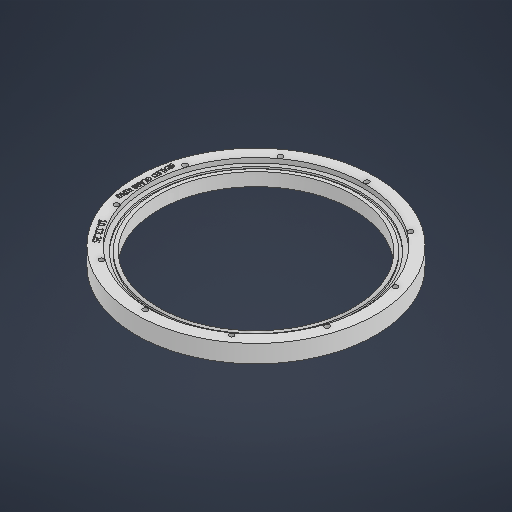
# Autodesk Inventor part: SealedGlassRing
Saved by Autodesk Inventor 2026.2 (Build 302298000, 298)
## iProperties
Created: 2025-06-19
Part Number: SealedGlassRing
Material: Generic
Document SubType Name: Modeling
Designer: mumin
Density: 1 g/cm^3
Appearance: Default
Author: mumin
Autodesk Inventor part; units mm, degrees
ref_plane "YZ Plane" through (0, 0, 0) normal (1, 0, 0) x (0, 1, 0)
ref_plane "XZ Plane" through (0, 0, 0) normal (0, 1, 0) x (-1, 0, 0)
ref_plane "XY Plane" through (0, 0, 0) normal (0, 0, 1) x (1, 0, 0)
sketch "Sketch1" plane through (0, 0, 0) normal (0, 1, 0) x (-1, 0, 0)
  circle A0 centre (0, 0) radius 110
  circle A1 centre (0, 0) radius 135
  dimension "d0" = 220
  dimension "d1" = 270
  constraints: 2 centre point, 2 coincident
  measures "d0" diameter of A0
  measures "d1" diameter of A1
extrude "Ring" add sketch "Sketch1" along normal blind 20
sketch "Sketch2" plane through (0, 20, 0) normal (0, 1, 0) x (1, 0, 0)
  circle A0 centre (0, 0) radius 122
  dimension "d4" = 244
  constraints: 1 centre point, 1 coincident
  measures "d4" diameter of A0
extrude "Glass Seat" cut sketch "Sketch2" against normal blind 5.3
sketch "Sketch3" plane through (0, 20, 0) normal (0, 1, 0) x (1, 0, 0)
  line L0 (0, 189) -> (0, -189) projected
  point P0 (0, 0)
  point P1 (0, 125)
  dimension "d14" = 125
  constraints: 1 point on line
  measures "d14" distance of point (0, 0) point (0, 125)
hole "Holes" at (0, 20, -125) direction (0, -1, 0) diameter 5.5 end through all
pattern_circular "Circular Pattern1" count 10 over 360 about axis through (0, -10, 0) along (0, 1, 0) of "Holes"
sketch "Sketch4" plane through (0, 20, 0) normal (0, 1, 0) x (1, 0, 0)
  line L0 (-123.4008, 33.078) -> (-123.4008, -40.8071) construction
  line L1 (-123.4008, -40.8071) -> (-126.5772, -40.8071) construction
  line L2 (-126.5772, -40.8071) -> (-126.5772, 33.078) construction
  line L3 (-126.5772, 33.078) -> (-123.4008, 33.078) construction
  spline S0 degree 2 poles (-128.5791, 31.1777) (-128.5791, 31.7207) (-128.3522, 32.4824) (-128.1901, 32.8187) knots 0 0 0 1 2 2 2
  line L4 (-128.1901, 32.8187) -> (-127.3554, 32.8187)
  line L5 (-127.3554, 32.8187) -> (-127.3554, 32.7701)
  spline S1 degree 2 poles (-127.3554, 32.7701) (-127.6634, 32.4419) (-128.0037, 31.6113) (-128.0037, 31.2263) knots 0 0 0 1 2 2 2
  spline S2 degree 2 poles (-128.0037, 31.2263) (-128.0037, 30.6753) (-127.5459, 30.1121) (-127.169, 30.1121) knots 0 0 0 1 2 2 2
  spline S3 degree 2 poles (-127.169, 30.1121) (-126.8692, 30.1121) (-126.4964, 30.4079) (-126.4032, 30.7279) knots 0 0 0 1 2 2 2
  spline S4 degree 2 poles (-126.4032, 30.7279) (-126.3384, 30.9589) (-126.2493, 31.3438) (-126.1763, 31.6315) knots 0 0 0 1 2 2 2
  spline S5 degree 2 poles (-126.1763, 31.6315) (-126.1074, 31.8908) (-125.9008, 32.3001) (-125.7347, 32.4581) knots 0 0 0 1 2 2 2
  spline S6 degree 2 poles (-125.7347, 32.4581) (-125.5685, 32.6121) (-125.1228, 32.7822) (-124.8311, 32.7822) knots 0 0 0 1 2 2 2
  spline S7 degree 2 poles (-124.8311, 32.7822) (-124.2233, 32.7822) (-123.4008, 31.8341) (-123.4008, 31.1007) knots 0 0 0 1 2 2 2
  spline S8 degree 2 poles (-123.4008, 31.1007) (-123.4008, 30.6793) (-123.5669, 29.9338) (-123.7249, 29.6137) knots 0 0 0 1 2 2 2
  line L6 (-123.7249, 29.6137) -> (-124.5191, 29.6137)
  line L7 (-124.5191, 29.6137) -> (-124.5191, 29.6623)
  spline S9 degree 2 poles (-124.5191, 29.6623) (-124.3003, 29.9014) (-123.9762, 30.6469) (-123.9762, 31.0561) knots 0 0 0 1 2 2 2
  spline S10 degree 2 poles (-123.9762, 31.0561) (-123.9762, 31.5181) (-124.4097, 32.0894) (-124.7622, 32.0894) knots 0 0 0 1 2 2 2
  spline S11 degree 2 poles (-124.7622, 32.0894) (-125.0783, 32.0894) (-125.4551, 31.7531) (-125.5402, 31.437) knots 0 0 0 1 2 2 2
  spline S12 degree 2 poles (-125.5402, 31.437) (-125.5969, 31.2263) (-125.7428, 30.6145) (-125.8036, 30.4119) knots 0 0 0 1 2 2 2
  spline S13 degree 2 poles (-125.8036, 30.4119) (-125.9616, 29.8973) (-126.5977, 29.4192) (-127.0637, 29.4192) knots 0 0 0 1 2 2 2
  spline S14 degree 2 poles (-127.0637, 29.4192) (-127.3595, 29.4192) (-127.9267, 29.6583) (-128.1253, 29.873) knots 0 0 0 1 2 2 2
  spline S15 degree 2 poles (-128.1253, 29.873) (-128.3441, 30.1121) (-128.5791, 30.7198) (-128.5791, 31.1777) knots 0 0 0 1 2 2 2
  line L8 (-128.4899, 28.7425) -> (-123.4899, 28.7425)
  line L9 (-123.4899, 28.7425) -> (-123.4899, 25.6145)
  line L10 (-123.4899, 25.6145) -> (-124.0815, 25.6145)
  line L11 (-124.0815, 25.6145) -> (-124.0815, 28.078)
  line L12 (-124.0815, 28.078) -> (-125.451, 28.078)
  line L13 (-125.451, 28.078) -> (-125.451, 25.7806)
  line L14 (-125.451, 25.7806) -> (-126.0426, 25.7806)
  line L15 (-126.0426, 25.7806) -> (-126.0426, 28.078)
  line L16 (-126.0426, 28.078) -> (-127.8984, 28.078)
  line L17 (-127.8984, 28.078) -> (-127.8984, 25.6145)
  line L18 (-127.8984, 25.6145) -> (-128.4899, 25.6145)
  line L19 (-128.4899, 25.6145) -> (-128.4899, 28.7425)
  line L20 (-128.4899, 25.4241) -> (-123.4899, 23.7385)
  line L21 (-123.4899, 23.7385) -> (-123.4899, 22.92)
  line L22 (-123.4899, 22.92) -> (-128.4899, 21.2344)
  line L23 (-128.4899, 21.2344) -> (-128.4899, 21.9354)
  line L24 (-128.4899, 21.9354) -> (-127.092, 22.3892)
  line L25 (-127.092, 22.3892) -> (-127.092, 24.2976)
  line L26 (-127.092, 24.2976) -> (-128.4899, 24.7514)
  line L27 (-128.4899, 24.7514) -> (-128.4899, 25.4241)
  line L28 (-126.5248, 22.5715) -> (-124.1707, 23.3455)
  line L29 (-124.1707, 23.3455) -> (-126.5248, 24.1153)
  line L30 (-126.5248, 24.1153) -> (-126.5248, 22.5715)
  line L31 (-128.4899, 17.8633) -> (-128.4899, 20.7604)
  line L32 (-128.4899, 20.7604) -> (-123.4899, 20.7604)
  line L33 (-123.4899, 20.7604) -> (-123.4899, 20.0959)
  line L34 (-123.4899, 20.0959) -> (-127.8984, 20.0959)
  line L35 (-127.8984, 20.0959) -> (-127.8984, 17.8633)
  line L36 (-127.8984, 17.8633) -> (-128.4899, 17.8633)
  line L37 (-128.4899, 17.3406) -> (-123.4899, 17.3406)
  line L38 (-123.4899, 17.3406) -> (-123.4899, 14.2126)
  line L39 (-123.4899, 14.2126) -> (-124.0815, 14.2126)
  line L40 (-124.0815, 14.2126) -> (-124.0815, 16.6761)
  line L41 (-124.0815, 16.6761) -> (-125.451, 16.6761)
  line L42 (-125.451, 16.6761) -> (-125.451, 14.3787)
  line L43 (-125.451, 14.3787) -> (-126.0426, 14.3787)
  line L44 (-126.0426, 14.3787) -> (-126.0426, 16.6761)
  line L45 (-126.0426, 16.6761) -> (-127.8984, 16.6761)
  line L46 (-127.8984, 16.6761) -> (-127.8984, 14.2126)
  line L47 (-127.8984, 14.2126) -> (-128.4899, 14.2126)
  line L48 (-128.4899, 14.2126) -> (-128.4899, 17.3406)
  spline S16 degree 2 poles (-125.994, 9.5408) (-126.6788, 9.5408) (-127.7809, 10.0959) (-128.0888, 10.5618) knots 0 0 0 1 2 2 2
  spline S17 degree 2 poles (-128.0888, 10.5618) (-128.3279, 10.9427) (-128.4899, 11.7247) (-128.4899, 12.3325) knots 0 0 0 1 2 2 2
  line L49 (-128.4899, 12.3325) -> (-128.4899, 13.4832)
  line L50 (-128.4899, 13.4832) -> (-123.4899, 13.4832)
  line L51 (-123.4899, 13.4832) -> (-123.4899, 12.3446)
  spline S18 degree 2 poles (-123.4899, 12.3446) (-123.4899, 11.6396) (-123.7006, 10.8373) (-123.887, 10.5537) knots 0 0 0 1 2 2 2
  spline S19 degree 2 poles (-123.887, 10.5537) (-124.2071, 10.0715) (-125.2647, 9.5408) (-125.994, 9.5408) knots 0 0 0 1 2 2 2
  spline S20 degree 2 poles (-125.9859, 10.2336) (-125.4105, 10.2336) (-124.5961, 10.6145) (-124.3651, 10.9913) knots 0 0 0 1 2 2 2
  spline S21 degree 2 poles (-124.3651, 10.9913) (-124.2071, 11.2587) (-124.0653, 11.8625) (-124.0653, 12.3122) knots 0 0 0 1 2 2 2
  line L52 (-124.0653, 12.3122) -> (-124.0653, 12.8187)
  line L53 (-124.0653, 12.8187) -> (-127.9146, 12.8187)
  line L54 (-127.9146, 12.8187) -> (-127.9146, 12.3122)
  spline S22 degree 2 poles (-127.9146, 12.3122) (-127.9146, 11.8706) (-127.7728, 11.202) (-127.5823, 10.9305) knots 0 0 0 1 2 2 2
  spline S23 degree 2 poles (-127.5823, 10.9305) (-127.3473, 10.5821) (-126.5694, 10.2336) (-125.9859, 10.2336) knots 0 0 0 1 2 2 2
  spline S24 degree 2 poles (-128.5872, 4.5772) (-128.5872, 5.108) (-128.263, 5.9873) (-127.9348, 6.3033) knots 0 0 0 1 2 2 2
  spline S25 degree 2 poles (-127.9348, 6.3033) (-127.6026, 6.6194) (-126.622, 6.9557) (-125.9859, 6.9557) knots 0 0 0 1 2 2 2
  spline S26 degree 2 poles (-125.9859, 6.9557) (-125.3822, 6.9557) (-124.4259, 6.6153) (-124.0856, 6.2993) knots 0 0 0 1 2 2 2
  spline S27 degree 2 poles (-124.0856, 6.2993) (-123.7574, 5.9954) (-123.4008, 5.104) (-123.4008, 4.5732) knots 0 0 0 1 2 2 2
  spline S28 degree 2 poles (-123.4008, 4.5732) (-123.4008, 4.3179) (-123.4737, 3.856) (-123.5386, 3.6453) knots 0 0 0 1 2 2 2
  spline S29 degree 2 poles (-123.5386, 3.6453) (-123.5872, 3.4751) (-123.7655, 3.0618) (-123.8303, 2.9362) knots 0 0 0 1 2 2 2
  line L55 (-123.8303, 2.9362) -> (-124.6326, 2.9362)
  line L56 (-124.6326, 2.9362) -> (-124.6326, 2.9929)
  spline S30 degree 2 poles (-124.6326, 2.9929) (-124.5232, 3.1185) (-124.3246, 3.3819) (-124.2112, 3.625) knots 0 0 0 1 2 2 2
  spline S31 degree 2 poles (-124.2112, 3.625) (-124.1099, 3.8276) (-123.9762, 4.3503) (-123.9762, 4.6502) knots 0 0 0 1 2 2 2
  spline S32 degree 2 poles (-123.9762, 4.6502) (-123.9762, 5.3714) (-125.0621, 6.2628) (-125.9656, 6.2628) knots 0 0 0 1 2 2 2
  spline S33 degree 2 poles (-125.9656, 6.2628) (-126.4681, 6.2628) (-127.2217, 6.0278) (-127.481, 5.8049) knots 0 0 0 1 2 2 2
  spline S34 degree 2 poles (-127.481, 5.8049) (-127.7403, 5.5902) (-128.0118, 4.9824) (-128.0118, 4.6015) knots 0 0 0 1 2 2 2
  spline S35 degree 2 poles (-128.0118, 4.6015) (-128.0118, 4.322) (-127.9308, 3.7628) (-127.8497, 3.5724) knots 0 0 0 1 2 2 2
  line L57 (-127.8497, 3.5724) -> (-126.5572, 3.5724)
  line L58 (-126.5572, 3.5724) -> (-126.5572, 4.7312)
  line L59 (-126.5572, 4.7312) -> (-125.9737, 4.7312)
  line L60 (-125.9737, 4.7312) -> (-125.9737, 2.916)
  line L61 (-125.9737, 2.916) -> (-128.1577, 2.916)
  spline S36 degree 2 poles (-128.1577, 2.916) (-128.2144, 3.0416) (-128.3886, 3.4711) (-128.4413, 3.6534) knots 0 0 0 1 2 2 2
  spline S37 degree 2 poles (-128.4413, 3.6534) (-128.5142, 3.9006) (-128.5872, 4.2976) (-128.5872, 4.5772) knots 0 0 0 1 2 2 2
  line L62 (-128.4899, -0.8158) -> (-128.4899, 2.0813)
  line L63 (-128.4899, 2.0813) -> (-123.4899, 2.0813)
  line L64 (-123.4899, 2.0813) -> (-123.4899, 1.4168)
  line L65 (-123.4899, 1.4168) -> (-127.8984, 1.4168)
  line L66 (-127.8984, 1.4168) -> (-127.8984, -0.8158)
  line L67 (-127.8984, -0.8158) -> (-128.4899, -0.8158)
  line L68 (-128.4899, -0.7996) -> (-123.4899, -2.4852)
  line L69 (-123.4899, -2.4852) -> (-123.4899, -3.3037)
  line L70 (-123.4899, -3.3037) -> (-128.4899, -4.9892)
  line L71 (-128.4899, -4.9892) -> (-128.4899, -4.2883)
  line L72 (-128.4899, -4.2883) -> (-127.092, -3.8345)
  line L73 (-127.092, -3.8345) -> (-127.092, -1.926)
  line L74 (-127.092, -1.926) -> (-128.4899, -1.4722)
  line L75 (-128.4899, -1.4722) -> (-128.4899, -0.7996)
  line L76 (-126.5248, -3.6521) -> (-124.1707, -2.8782)
  line L77 (-124.1707, -2.8782) -> (-126.5248, -2.1084)
  line L78 (-126.5248, -2.1084) -> (-126.5248, -3.6521)
  spline S38 degree 2 poles (-128.5791, -6.8571) (-128.5791, -6.3142) (-128.3522, -5.5524) (-128.1901, -5.2161) knots 0 0 0 1 2 2 2
  line L79 (-128.1901, -5.2161) -> (-127.3554, -5.2161)
  line L80 (-127.3554, -5.2161) -> (-127.3554, -5.2648)
  spline S39 degree 2 poles (-127.3554, -5.2648) (-127.6634, -5.593) (-128.0037, -6.4236) (-128.0037, -6.8085) knots 0 0 0 1 2 2 2
  spline S40 degree 2 poles (-128.0037, -6.8085) (-128.0037, -7.3596) (-127.5459, -7.9228) (-127.169, -7.9228) knots 0 0 0 1 2 2 2
  spline S41 degree 2 poles (-127.169, -7.9228) (-126.8692, -7.9228) (-126.4964, -7.627) (-126.4032, -7.3069) knots 0 0 0 1 2 2 2
  spline S42 degree 2 poles (-126.4032, -7.3069) (-126.3384, -7.0759) (-126.2493, -6.691) (-126.1763, -6.4033) knots 0 0 0 1 2 2 2
  spline S43 degree 2 poles (-126.1763, -6.4033) (-126.1074, -6.144) (-125.9008, -5.7348) (-125.7347, -5.5768) knots 0 0 0 1 2 2 2
  spline S44 degree 2 poles (-125.7347, -5.5768) (-125.5685, -5.4228) (-125.1228, -5.2526) (-124.8311, -5.2526) knots 0 0 0 1 2 2 2
  spline S45 degree 2 poles (-124.8311, -5.2526) (-124.2233, -5.2526) (-123.4008, -6.2007) (-123.4008, -6.9341) knots 0 0 0 1 2 2 2
  spline S46 degree 2 poles (-123.4008, -6.9341) (-123.4008, -7.3555) (-123.5669, -8.1011) (-123.7249, -8.4212) knots 0 0 0 1 2 2 2
  line L81 (-123.7249, -8.4212) -> (-124.5191, -8.4212)
  line L82 (-124.5191, -8.4212) -> (-124.5191, -8.3725)
  spline S47 degree 2 poles (-124.5191, -8.3725) (-124.3003, -8.1335) (-123.9762, -7.3879) (-123.9762, -6.9787) knots 0 0 0 1 2 2 2
  spline S48 degree 2 poles (-123.9762, -6.9787) (-123.9762, -6.5168) (-124.4097, -5.9455) (-124.7622, -5.9455) knots 0 0 0 1 2 2 2
  spline S49 degree 2 poles (-124.7622, -5.9455) (-125.0783, -5.9455) (-125.4551, -6.2818) (-125.5402, -6.5978) knots 0 0 0 1 2 2 2
  spline S50 degree 2 poles (-125.5402, -6.5978) (-125.5969, -6.8085) (-125.7428, -7.4203) (-125.8036, -7.6229) knots 0 0 0 1 2 2 2
  spline S51 degree 2 poles (-125.8036, -7.6229) (-125.9616, -8.1375) (-126.5977, -8.6156) (-127.0637, -8.6156) knots 0 0 0 1 2 2 2
  spline S52 degree 2 poles (-127.0637, -8.6156) (-127.3595, -8.6156) (-127.9267, -8.3766) (-128.1253, -8.1618) knots 0 0 0 1 2 2 2
  spline S53 degree 2 poles (-128.1253, -8.1618) (-128.3441, -7.9228) (-128.5791, -7.315) (-128.5791, -6.8571) knots 0 0 0 1 2 2 2
  spline S54 degree 2 poles (-128.5791, -10.6862) (-128.5791, -10.1432) (-128.3522, -9.3815) (-128.1901, -9.0451) knots 0 0 0 1 2 2 2
  line L83 (-128.1901, -9.0451) -> (-127.3554, -9.0451)
  line L84 (-127.3554, -9.0451) -> (-127.3554, -9.0938)
  spline S55 degree 2 poles (-127.3554, -9.0938) (-127.6634, -9.422) (-128.0037, -10.2526) (-128.0037, -10.6375) knots 0 0 0 1 2 2 2
  spline S56 degree 2 poles (-128.0037, -10.6375) (-128.0037, -11.1886) (-127.5459, -11.7518) (-127.169, -11.7518) knots 0 0 0 1 2 2 2
  spline S57 degree 2 poles (-127.169, -11.7518) (-126.8692, -11.7518) (-126.4964, -11.456) (-126.4032, -11.1359) knots 0 0 0 1 2 2 2
  spline S58 degree 2 poles (-126.4032, -11.1359) (-126.3384, -10.905) (-126.2493, -10.52) (-126.1763, -10.2323) knots 0 0 0 1 2 2 2
  spline S59 degree 2 poles (-126.1763, -10.2323) (-126.1074, -9.973) (-125.9008, -9.5638) (-125.7347, -9.4058) knots 0 0 0 1 2 2 2
  spline S60 degree 2 poles (-125.7347, -9.4058) (-125.5685, -9.2518) (-125.1228, -9.0816) (-124.8311, -9.0816) knots 0 0 0 1 2 2 2
  spline S61 degree 2 poles (-124.8311, -9.0816) (-124.2233, -9.0816) (-123.4008, -10.0298) (-123.4008, -10.7631) knots 0 0 0 1 2 2 2
  spline S62 degree 2 poles (-123.4008, -10.7631) (-123.4008, -11.1845) (-123.5669, -11.9301) (-123.7249, -12.2502) knots 0 0 0 1 2 2 2
  line L85 (-123.7249, -12.2502) -> (-124.5191, -12.2502)
  line L86 (-124.5191, -12.2502) -> (-124.5191, -12.2015)
  spline S63 degree 2 poles (-124.5191, -12.2015) (-124.3003, -11.9625) (-123.9762, -11.2169) (-123.9762, -10.8077) knots 0 0 0 1 2 2 2
  spline S64 degree 2 poles (-123.9762, -10.8077) (-123.9762, -10.3458) (-124.4097, -9.7745) (-124.7622, -9.7745) knots 0 0 0 1 2 2 2
  spline S65 degree 2 poles (-124.7622, -9.7745) (-125.0783, -9.7745) (-125.4551, -10.1108) (-125.5402, -10.4268) knots 0 0 0 1 2 2 2
  spline S66 degree 2 poles (-125.5402, -10.4268) (-125.5969, -10.6375) (-125.7428, -11.2494) (-125.8036, -11.452) knots 0 0 0 1 2 2 2
  spline S67 degree 2 poles (-125.8036, -11.452) (-125.9616, -11.9665) (-126.5977, -12.4447) (-127.0637, -12.4447) knots 0 0 0 1 2 2 2
  spline S68 degree 2 poles (-127.0637, -12.4447) (-127.3595, -12.4447) (-127.9267, -12.2056) (-128.1253, -11.9909) knots 0 0 0 1 2 2 2
  spline S69 degree 2 poles (-128.1253, -11.9909) (-128.3441, -11.7518) (-128.5791, -11.144) (-128.5791, -10.6862) knots 0 0 0 1 2 2 2
  line L87 (-128.4899, -19.1383) -> (-128.4899, -18.2753)
  line L88 (-128.4899, -18.2753) -> (-126.5005, -16.6951)
  line L89 (-126.5005, -16.6951) -> (-126.5005, -15.9333)
  line L90 (-126.5005, -15.9333) -> (-128.4899, -15.9333)
  line L91 (-128.4899, -15.9333) -> (-128.4899, -15.2688)
  line L92 (-128.4899, -15.2688) -> (-123.4899, -15.2688)
  line L93 (-123.4899, -15.2688) -> (-123.4899, -16.5573)
  spline S70 degree 2 poles (-123.4899, -16.5573) (-123.4899, -16.9868) (-123.5831, -17.5662) (-123.7533, -17.8296) knots 0 0 0 1 2 2 2
  spline S71 degree 2 poles (-123.7533, -17.8296) (-123.9235, -18.093) (-124.4543, -18.3968) (-124.8473, -18.3968) knots 0 0 0 1 2 2 2
  spline S72 degree 2 poles (-124.8473, -18.3968) (-125.3943, -18.3968) (-126.1358, -17.8377) (-126.3141, -17.3596) knots 0 0 0 1 2 2 2
  line L94 (-126.3141, -17.3596) -> (-128.4899, -19.1383)
  spline S73 degree 2 poles (-124.9, -17.704) (-124.6812, -17.704) (-124.3449, -17.55) (-124.2355, -17.3879) knots 0 0 0 1 2 2 2
  spline S74 degree 2 poles (-124.2355, -17.3879) (-124.1423, -17.2461) (-124.0653, -16.8693) (-124.0653, -16.5938) knots 0 0 0 1 2 2 2
  line L95 (-124.0653, -16.5938) -> (-124.0653, -15.9333)
  line L96 (-124.0653, -15.9333) -> (-125.9454, -15.9333)
  line L97 (-125.9454, -15.9333) -> (-125.9454, -16.5168)
  spline S75 degree 2 poles (-125.9454, -16.5168) (-125.9454, -16.8045) (-125.8441, -17.2623) (-125.686, -17.4203) knots 0 0 0 1 2 2 2
  spline S76 degree 2 poles (-125.686, -17.4203) (-125.5483, -17.5662) (-125.1593, -17.704) (-124.9, -17.704) knots 0 0 0 1 2 2 2
  line L98 (-128.4899, -21.2777) -> (-128.4899, -19.3409)
  line L99 (-128.4899, -19.3409) -> (-127.9794, -19.3409)
  line L100 (-127.9794, -19.3409) -> (-127.9794, -19.9771)
  line L101 (-127.9794, -19.9771) -> (-124.0005, -19.9771)
  line L102 (-124.0005, -19.9771) -> (-124.0005, -19.3409)
  line L103 (-124.0005, -19.3409) -> (-123.4899, -19.3409)
  line L104 (-123.4899, -19.3409) -> (-123.4899, -21.2777)
  line L105 (-123.4899, -21.2777) -> (-124.0005, -21.2777)
  line L106 (-124.0005, -21.2777) -> (-124.0005, -20.6416)
  line L107 (-124.0005, -20.6416) -> (-127.9794, -20.6416)
  line L108 (-127.9794, -20.6416) -> (-127.9794, -21.2777)
  line L109 (-127.9794, -21.2777) -> (-128.4899, -21.2777)
  line L110 (-128.4899, -25.678) -> (-128.4899, -24.9325)
  line L111 (-128.4899, -24.9325) -> (-124.1788, -22.7202)
  line L112 (-124.1788, -22.7202) -> (-128.4899, -22.7202)
  line L113 (-128.4899, -22.7202) -> (-128.4899, -22.1003)
  line L114 (-128.4899, -22.1003) -> (-123.4899, -22.1003)
  line L115 (-123.4899, -22.1003) -> (-123.4899, -23.0443)
  line L116 (-123.4899, -23.0443) -> (-127.4486, -25.0581)
  line L117 (-127.4486, -25.0581) -> (-123.4899, -25.0581)
  line L118 (-123.4899, -25.0581) -> (-123.4899, -25.678)
  line L119 (-123.4899, -25.678) -> (-128.4899, -25.678)
  spline S77 degree 2 poles (-128.5872, -28.7858) (-128.5872, -28.255) (-128.263, -27.3758) (-127.9348, -27.0597) knots 0 0 0 1 2 2 2
  spline S78 degree 2 poles (-127.9348, -27.0597) (-127.6026, -26.7437) (-126.622, -26.4074) (-125.9859, -26.4074) knots 0 0 0 1 2 2 2
  spline S79 degree 2 poles (-125.9859, -26.4074) (-125.3822, -26.4074) (-124.4259, -26.7477) (-124.0856, -27.0638) knots 0 0 0 1 2 2 2
  spline S80 degree 2 poles (-124.0856, -27.0638) (-123.7574, -27.3677) (-123.4008, -28.2591) (-123.4008, -28.7899) knots 0 0 0 1 2 2 2
  spline S81 degree 2 poles (-123.4008, -28.7899) (-123.4008, -29.0451) (-123.4737, -29.5071) (-123.5386, -29.7178) knots 0 0 0 1 2 2 2
  spline S82 degree 2 poles (-123.5386, -29.7178) (-123.5872, -29.8879) (-123.7655, -30.3012) (-123.8303, -30.4268) knots 0 0 0 1 2 2 2
  line L120 (-123.8303, -30.4268) -> (-124.6326, -30.4268)
  line L121 (-124.6326, -30.4268) -> (-124.6326, -30.3701)
  spline S83 degree 2 poles (-124.6326, -30.3701) (-124.5232, -30.2445) (-124.3246, -29.9811) (-124.2112, -29.738) knots 0 0 0 1 2 2 2
  spline S84 degree 2 poles (-124.2112, -29.738) (-124.1099, -29.5354) (-123.9762, -29.0127) (-123.9762, -28.7129) knots 0 0 0 1 2 2 2
  spline S85 degree 2 poles (-123.9762, -28.7129) (-123.9762, -27.9917) (-125.0621, -27.1003) (-125.9656, -27.1003) knots 0 0 0 1 2 2 2
  spline S86 degree 2 poles (-125.9656, -27.1003) (-126.4681, -27.1003) (-127.2217, -27.3353) (-127.481, -27.5581) knots 0 0 0 1 2 2 2
  spline S87 degree 2 poles (-127.481, -27.5581) (-127.7403, -27.7729) (-128.0118, -28.3806) (-128.0118, -28.7615) knots 0 0 0 1 2 2 2
  spline S88 degree 2 poles (-128.0118, -28.7615) (-128.0118, -29.0411) (-127.9308, -29.6003) (-127.8497, -29.7907) knots 0 0 0 1 2 2 2
  line L122 (-127.8497, -29.7907) -> (-126.5572, -29.7907)
  line L123 (-126.5572, -29.7907) -> (-126.5572, -28.6319)
  line L124 (-126.5572, -28.6319) -> (-125.9737, -28.6319)
  line L125 (-125.9737, -28.6319) -> (-125.9737, -30.4471)
  line L126 (-125.9737, -30.4471) -> (-128.1577, -30.4471)
  spline S89 degree 2 poles (-128.1577, -30.4471) (-128.2144, -30.3215) (-128.3886, -29.892) (-128.4413, -29.7097) knots 0 0 0 1 2 2 2
  spline S90 degree 2 poles (-128.4413, -29.7097) (-128.5142, -29.4625) (-128.5872, -29.0654) (-128.5872, -28.7858) knots 0 0 0 1 2 2 2
  point P0 (0, 0)
  constraints: 2 other
emboss "LABEL" sketch "Sketch4" operation cut depth 1 direction (0, -1, 0)
sketch "Sketch6" plane through (0, 20, 0) normal (0, 1, 0) x (1, 0, 0)
  line L0 (-109.3924, -58.9981) -> (-94.816, -80.0727) construction
  line L1 (-94.816, -80.0727) -> (-101.766, -84.8798) construction
  line L2 (-101.766, -84.8798) -> (-116.3425, -63.8052) construction
  line L3 (-116.3425, -63.8052) -> (-109.3924, -58.9981) construction
  line L4 (-112.2488, -65.6382) -> (-113.9138, -63.2309)
  line L5 (-113.9138, -63.2309) -> (-113.4099, -62.8824)
  line L6 (-113.4099, -62.8824) -> (-112.7904, -63.7782)
  line L7 (-112.7904, -63.7782) -> (-109.4833, -61.4908)
  line L8 (-109.4833, -61.4908) -> (-110.1029, -60.595)
  line L9 (-110.1029, -60.595) -> (-109.651, -60.2825)
  spline S0 degree 2 poles (-109.651, -60.2825) (-109.2997, -60.7903) (-108.6799, -61.0711) (-108.2579, -60.8265) knots 0 0 0 1 2 2 2
  line L10 (-108.2579, -60.8265) -> (-107.9038, -61.3383)
  line L11 (-107.9038, -61.3383) -> (-112.3506, -64.414)
  line L12 (-112.3506, -64.414) -> (-111.7449, -65.2897)
  line L13 (-111.7449, -65.2897) -> (-112.2488, -65.6382)
  spline S1 degree 2 poles (-107.0294, -67.9106) (-108.357, -68.8289) (-110.1345, -68.9173) (-110.6904, -68.1135) knots 0 0 0 1 2 2 2
  spline S2 degree 2 poles (-110.6904, -68.1135) (-111.2547, -67.2977) (-110.5153, -65.6571) (-109.2157, -64.7582) knots 0 0 0 1 2 2 2
  spline S3 degree 2 poles (-109.2157, -64.7582) (-107.88, -63.8344) (-106.1105, -63.7516) (-105.5518, -64.5593) knots 0 0 0 1 2 2 2
  spline S4 degree 2 poles (-105.5518, -64.5593) (-104.9904, -65.3711) (-105.7417, -67.02) (-107.0294, -67.9106) knots 0 0 0 1 2 2 2
  spline S5 degree 2 poles (-109.1193, -68.1028) (-108.809, -68.0301) (-108.0019, -67.5901) (-107.494, -67.2388) knots 0 0 0 1 2 2 2
  spline S6 degree 2 poles (-107.494, -67.2388) (-106.9862, -66.8875) (-106.2937, -66.2903) (-106.1109, -66.0161) knots 0 0 0 1 2 2 2
  spline S7 degree 2 poles (-106.1109, -66.0161) (-105.9281, -65.7419) (-105.9088, -65.2142) (-106.0997, -64.9383) knots 0 0 0 1 2 2 2
  spline S8 degree 2 poles (-106.0997, -64.9383) (-106.2905, -64.6623) (-106.7966, -64.4862) (-107.1285, -64.562) knots 0 0 0 1 2 2 2
  spline S9 degree 2 poles (-107.1285, -64.562) (-107.4495, -64.6363) (-108.2671, -65.0954) (-108.751, -65.4301) knots 0 0 0 1 2 2 2
  spline S10 degree 2 poles (-108.751, -65.4301) (-109.2708, -65.7896) (-109.9224, -66.3349) (-110.1224, -66.6269) knots 0 0 0 1 2 2 2
  spline S11 degree 2 poles (-110.1224, -66.6269) (-110.312, -66.8999) (-110.3417, -67.4467) (-110.1426, -67.7346) knots 0 0 0 1 2 2 2
  spline S12 degree 2 poles (-110.1426, -67.7346) (-109.9545, -68.0065) (-109.4484, -68.1826) (-109.1193, -68.1028) knots 0 0 0 1 2 2 2
  line L14 (-108.3267, -71.3087) -> (-108.8744, -70.5169)
  line L15 (-108.8744, -70.5169) -> (-107.9306, -69.8642)
  line L16 (-107.9306, -69.8642) -> (-107.383, -70.6559)
  line L17 (-107.383, -70.6559) -> (-108.3267, -71.3087)
  line L18 (-105.7047, -75.0997) -> (-107.3697, -72.6923)
  line L19 (-107.3697, -72.6923) -> (-106.8659, -72.3438)
  line L20 (-106.8659, -72.3438) -> (-106.2463, -73.2396)
  line L21 (-106.2463, -73.2396) -> (-102.9392, -70.9522)
  line L22 (-102.9392, -70.9522) -> (-103.5588, -70.0564)
  line L23 (-103.5588, -70.0564) -> (-103.1069, -69.7439)
  spline S13 degree 2 poles (-103.1069, -69.7439) (-102.7556, -70.2518) (-102.1358, -70.5325) (-101.7138, -70.2879) knots 0 0 0 1 2 2 2
  line L24 (-101.7138, -70.2879) -> (-101.3598, -70.7997)
  line L25 (-101.3598, -70.7997) -> (-105.8065, -73.8754)
  line L26 (-105.8065, -73.8754) -> (-105.2008, -74.7512)
  line L27 (-105.2008, -74.7512) -> (-105.7047, -75.0997)
  spline S14 degree 2 poles (-99.689, -74.2496) (-99.8135, -74.0696) (-100.1476, -73.7746) (-100.3345, -73.6496) knots 0 0 0 1 2 2 2
  spline S15 degree 2 poles (-100.3345, -73.6496) (-100.5131, -73.5367) (-100.8203, -73.4003) (-100.9479, -73.3526) knots 0 0 0 1 2 2 2
  line L28 (-100.9479, -73.3526) -> (-100.9755, -73.3126)
  line L29 (-100.9755, -73.3126) -> (-100.2757, -72.8286)
  spline S16 degree 2 poles (-100.2757, -72.8286) (-100.0104, -72.9643) (-99.3108, -73.5741) (-99.0812, -73.906) knots 0 0 0 1 2 2 2
  spline S17 degree 2 poles (-99.0812, -73.906) (-98.8489, -74.2419) (-98.6391, -74.8358) (-98.642, -75.1394) knots 0 0 0 1 2 2 2
  spline S18 degree 2 poles (-98.642, -75.1394) (-98.6486, -75.4632) (-98.9456, -75.9996) (-99.2495, -76.2099) knots 0 0 0 1 2 2 2
  spline S19 degree 2 poles (-99.2495, -76.2099) (-99.6574, -76.492) (-100.6439, -76.3821) (-100.9838, -76.0615) knots 0 0 0 1 2 2 2
  line L30 (-100.9838, -76.0615) -> (-101.0318, -76.0947)
  spline S20 degree 2 poles (-101.0318, -76.0947) (-100.9559, -76.2728) (-100.8537, -76.7282) (-100.8926, -76.9798) knots 0 0 0 1 2 2 2
  spline S21 degree 2 poles (-100.8926, -76.9798) (-100.9275, -77.2285) (-101.2426, -77.7303) (-101.5665, -77.9543) knots 0 0 0 1 2 2 2
  spline S22 degree 2 poles (-101.5665, -77.9543) (-101.8984, -78.1839) (-102.6199, -78.3459) (-102.9797, -78.2873) knots 0 0 0 1 2 2 2
  spline S23 degree 2 poles (-102.9797, -78.2873) (-103.353, -78.2263) (-104.0081, -77.7749) (-104.2764, -77.387) knots 0 0 0 1 2 2 2
  spline S24 degree 2 poles (-104.2764, -77.387) (-104.5336, -77.0151) (-104.857, -76.1628) (-104.9045, -75.8291) knots 0 0 0 1 2 2 2
  line L31 (-104.9045, -75.8291) -> (-104.2047, -75.3451)
  line L32 (-104.2047, -75.3451) -> (-104.1715, -75.3931)
  spline S25 degree 2 poles (-104.1715, -75.3931) (-104.1797, -75.7061) (-103.9728, -76.6036) (-103.7322, -76.9515) knots 0 0 0 1 2 2 2
  spline S26 degree 2 poles (-103.7322, -76.9515) (-103.5911, -77.1554) (-103.181, -77.4748) (-102.939, -77.5084) knots 0 0 0 1 2 2 2
  spline S27 degree 2 poles (-102.939, -77.5084) (-102.6998, -77.538) (-102.2511, -77.4346) (-101.9832, -77.2493) knots 0 0 0 1 2 2 2
  spline S28 degree 2 poles (-101.9832, -77.2493) (-101.7152, -77.064) (-101.4752, -76.6674) (-101.472, -76.4583) knots 0 0 0 1 2 2 2
  spline S29 degree 2 poles (-101.472, -76.4583) (-101.4689, -76.2492) (-101.6556, -75.8167) (-101.8105, -75.5928) knots 0 0 0 1 2 2 2
  line L33 (-101.8105, -75.5928) -> (-102.0041, -75.3129)
  line L34 (-102.0041, -75.3129) -> (-101.4563, -74.9339)
  line L35 (-101.4563, -74.9339) -> (-101.3042, -75.1539)
  spline S30 degree 2 poles (-101.3042, -75.1539) (-100.9972, -75.5977) (-100.186, -75.8644) (-99.7822, -75.5851) knots 0 0 0 1 2 2 2
  spline S31 degree 2 poles (-99.7822, -75.5851) (-99.5942, -75.4551) (-99.4259, -75.1258) (-99.4261, -74.9545) knots 0 0 0 1 2 2 2
  spline S32 degree 2 poles (-99.4261, -74.9545) (-99.4279, -74.7725) (-99.5701, -74.4215) (-99.689, -74.2496) knots 0 0 0 1 2 2 2
  line L36 (-101.7827, -80.7701) -> (-102.3303, -79.9783)
  line L37 (-102.3303, -79.9783) -> (-101.3866, -79.3256)
  line L38 (-101.3866, -79.3256) -> (-100.8389, -80.1174)
  line L39 (-100.8389, -80.1174) -> (-101.7827, -80.7701)
  line L40 (-98.9891, -84.809) -> (-101.094, -81.7658)
  line L41 (-101.094, -81.7658) -> (-100.3942, -81.2818)
  spline S33 degree 2 poles (-100.3942, -81.2818) (-99.8594, -81.3967) (-98.8838, -81.5851) (-98.3822, -81.652) knots 0 0 0 1 2 2 2
  spline S34 degree 2 poles (-98.3822, -81.652) (-97.3724, -81.7872) (-96.3437, -81.6846) (-95.9479, -81.4108) knots 0 0 0 1 2 2 2
  spline S35 degree 2 poles (-95.9479, -81.4108) (-95.7399, -81.2669) (-95.5165, -80.9232) (-95.4967, -80.7381) knots 0 0 0 1 2 2 2
  spline S36 degree 2 poles (-95.4967, -80.7381) (-95.477, -80.553) (-95.5872, -80.1799) (-95.7144, -79.996) knots 0 0 0 1 2 2 2
  spline S37 degree 2 poles (-95.7144, -79.996) (-95.8361, -79.82) (-96.173, -79.521) (-96.3544, -79.4041) knots 0 0 0 1 2 2 2
  spline S38 degree 2 poles (-96.3544, -79.4041) (-96.5072, -79.3028) (-96.847, -79.1535) (-96.9583, -79.1123) knots 0 0 0 1 2 2 2
  line L42 (-96.9583, -79.1123) -> (-96.9832, -79.0763)
  line L43 (-96.9832, -79.0763) -> (-96.2793, -78.5895)
  spline S39 degree 2 poles (-96.2793, -78.5895) (-96.0383, -78.7243) (-95.3362, -79.3205) (-95.1094, -79.6485) knots 0 0 0 1 2 2 2
  spline S40 degree 2 poles (-95.1094, -79.6485) (-94.6309, -80.3403) (-94.8234, -81.6262) (-95.4472, -82.0577) knots 0 0 0 1 2 2 2
  spline S41 degree 2 poles (-95.4472, -82.0577) (-95.7391, -82.2596) (-96.321, -82.4611) (-96.6119, -82.4849) knots 0 0 0 1 2 2 2
  spline S42 degree 2 poles (-96.6119, -82.4849) (-96.9109, -82.5143) (-97.5754, -82.4596) (-97.9121, -82.4087) knots 0 0 0 1 2 2 2
  spline S43 degree 2 poles (-97.9121, -82.4087) (-98.4677, -82.3319) (-99.7238, -82.0715) (-100.0934, -81.9901) knots 0 0 0 1 2 2 2
  line L44 (-100.0934, -81.9901) -> (-98.4173, -84.4135)
  line L45 (-98.4173, -84.4135) -> (-98.9891, -84.809)
  spline S44 degree 2 poles (-94.8963, -87.3758) (-95.2522, -87.6219) (-96.0177, -87.8144) (-96.3855, -87.7614) knots 0 0 0 1 2 2 2
  spline S45 degree 2 poles (-96.3855, -87.7614) (-96.7532, -87.7083) (-97.4419, -87.2683) (-97.7074, -86.8844) knots 0 0 0 1 2 2 2
  spline S46 degree 2 poles (-97.7074, -86.8844) (-97.9508, -86.5325) (-98.2706, -85.7368) (-98.3209, -85.3991) knots 0 0 0 1 2 2 2
  line L46 (-98.3209, -85.3991) -> (-97.621, -84.9151)
  line L47 (-97.621, -84.9151) -> (-97.5879, -84.9631)
  spline S47 degree 2 poles (-97.5879, -84.9631) (-97.5913, -85.0778) (-97.5389, -85.4613) (-97.4839, -85.6775) knots 0 0 0 1 2 2 2
  spline S48 degree 2 poles (-97.4839, -85.6775) (-97.4164, -85.9204) (-97.2683, -86.2969) (-97.1273, -86.5008) knots 0 0 0 1 2 2 2
  spline S49 degree 2 poles (-97.1273, -86.5008) (-96.989, -86.7008) (-96.585, -86.9771) (-96.335, -87.0052) knots 0 0 0 1 2 2 2
  spline S50 degree 2 poles (-96.335, -87.0052) (-96.1013, -87.0268) (-95.6209, -86.8838) (-95.357, -86.7012) knots 0 0 0 1 2 2 2
  spline S51 degree 2 poles (-95.357, -86.7012) (-95.0931, -86.5187) (-94.8567, -86.1424) (-94.8388, -85.929) knots 0 0 0 1 2 2 2
  spline S52 degree 2 poles (-94.8388, -85.929) (-94.8116, -85.7032) (-94.9953, -85.2154) (-95.1696, -84.9635) knots 0 0 0 1 2 2 2
  spline S53 degree 2 poles (-95.1696, -84.9635) (-95.3576, -84.6916) (-95.815, -84.2098) (-95.9644, -84.0708) knots 0 0 0 1 2 2 2
  line L48 (-95.9644, -84.0708) -> (-93.4211, -82.3117)
  line L49 (-93.4211, -82.3117) -> (-91.5486, -85.0189)
  line L50 (-91.5486, -85.0189) -> (-92.1284, -85.42)
  line L51 (-92.1284, -85.42) -> (-93.5612, -83.3485)
  line L52 (-93.5612, -83.3485) -> (-94.8768, -84.2585)
  spline S54 degree 2 poles (-94.8768, -84.2585) (-94.7778, -84.3674) (-94.6054, -84.5911) (-94.539, -84.687) knots 0 0 0 1 2 2 2
  spline S55 degree 2 poles (-94.539, -84.687) (-94.2763, -85.0669) (-94.0379, -85.6765) (-94.0559, -86.0437) knots 0 0 0 1 2 2 2
  spline S56 degree 2 poles (-94.0559, -86.0437) (-94.0711, -86.4149) (-94.4484, -87.066) (-94.8963, -87.3758) knots 0 0 0 1 2 2 2
  point P0 (0, 0)
  constraints: 2 other
emboss "DATE" sketch "Sketch6" operation cut depth 1 direction (0, -1, 0)
sketch "Sketch7" plane through (0, 0, 0) normal (0, 0, 1) x (1, 0, 0)
  line L0 (110, 14.7) -> (-110, 14.7) projected
  line L1 (-122, 14.7) -> (122, 14.7) projected
  line L2 (114, 14.7) -> (117, 14.7)
  line L3 (117, 14.7) -> (117, 12.7)
  line L4 (117, 12.7) -> (114, 12.7)
  line L5 (114, 12.7) -> (114, 14.7)
  line L6 (0, -2.94) -> (0, 17.64) projected
  line L7 (135, 0) -> (-135, 0) projected
  line L8 (117, 0) -> (114, 0)
  line L9 (114, 0) -> (114, 2.5)
  line L10 (114, 2.5) -> (117, 2.5)
  line L11 (117, 2.5) -> (117, 0)
  point P0 (0, 0)
  dimension "d29" = 3
  dimension "d30" = 2
  dimension "d31" = 114
  dimension "d33" = 3
  dimension "d34" = 2.5
  constraints: 16 end point, 4 parallel, 2 horizontal, 2 perpendicular, 2 point on line
  measures "d29" distance of L3.end L4.end
  measures "d30" distance of L2.end L3.end
  measures "d31" distance from line of point (0, 0) L5
  measures "d33" distance of L9.end L10.end
  measures "d34" distance of L8.end L9.end
revolve "Seal Grooves" cut sketch "Sketch7" angle 360 about axis through (0, -10, 0) along (0, 1, 0)
body "Solid1"
